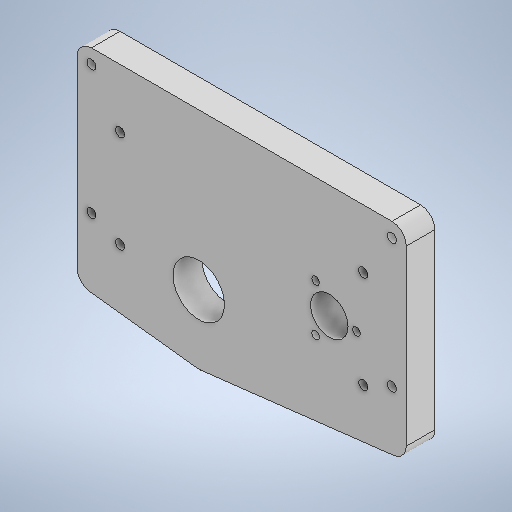
# Autodesk Inventor part: small_plate_motor
Saved by Autodesk Inventor 2025.1 (Build 291241000, 241)
## iProperties
Created: 2024-12-20
Part Number: small_plate_motor
Material: 一般
Document SubType Name: Modeling
Designer: yuki0520
Density: 1 g/cm^3
Appearance: 既定
Author: yuki0520
Autodesk Inventor part; units mm, degrees
ref_plane "YZ Plane" through (0, 0, 0) normal (1, 0, 0) x (0, 1, 0)
ref_plane "XZ Plane" through (0, 0, 0) normal (0, 1, 0) x (-1, 0, 0)
ref_plane "XY Plane" through (0, 0, 0) normal (0, 0, 1) x (1, 0, 0)
sketch "スケッチ1" plane through (0, 0, 0) normal (0, 0, 1) x (1, 0, 0)
  point P0 (0, 0)
sketch "スケッチ2" plane through (0, 0, 0) normal (0, 0, 1) x (1, 0, 0)
  line L0 (72.5, -37.5) -> (-72.5, -37.5)
  line L1 (-72.5, -37.5) -> (-72.5, 37.5)
  line L2 (-72.5, 37.5) -> (72.5, 37.5)
  line L3 (72.5, 37.5) -> (72.5, -37.5)
  line L4 (72.5, -37.5) -> (-72.5, 37.5) construction
  line L5 (-72.5, -37.5) -> (72.5, 37.5) construction
  circle A0 centre (-48, -17) radius 6.05
  circle A1 centre (-48, -17) radius 9
  circle A2 centre (-57, -17) radius 1.6
  circle A3 centre (-48, -26) radius 1.6
  circle A4 centre (-39, -17) radius 1.6
  circle A5 centre (-48, -8) radius 1.6
  line L6 (67.5, 32.5) -> (-67.5, 32.5)
  line L7 (-67.5, 32.5) -> (-67.5, -32.5)
  line L8 (-67.5, -32.5) -> (67.5, -32.5)
  line L9 (67.5, -32.5) -> (67.5, 32.5)
  line L10 (-67.5, 32.5) -> (-67.5, 12.5) construction
  line L11 (-69.1, 32.5) -> (-69.1, 12.5)
  line L12 (-65.9, 12.5) -> (-65.9, 32.5)
  arc A6 (-65.9, 32.5) -> (-69.1, 32.5) centre (-67.5, 32.5) ccw
  arc A7 (-69.1, 12.5) -> (-65.9, 12.5) centre (-67.5, 12.5) ccw
  line L13 (-67.5, 32.5) -> (-47.5, 32.5) construction
  line L14 (-67.5, -32.5) -> (-67.5, -12.5) construction
  line L15 (-65.9, -32.5) -> (-65.9, -12.5)
  line L16 (-69.1, -12.5) -> (-69.1, -32.5)
  arc A8 (-69.1, -32.5) -> (-65.9, -32.5) centre (-67.5, -32.5) ccw
  arc A9 (-65.9, -12.5) -> (-69.1, -12.5) centre (-67.5, -12.5) ccw
  line L17 (-67.5, -32.5) -> (-47.5, -32.5) construction
  line L18 (67.5, 32.5) -> (105, 32.5) construction
  line L19 (-72.5, -17) -> (72.5, -17)
  circle A10 centre (0, -17) radius 9
  circle A11 centre (0, -17) radius 39
  line L20 (-65, 37.5) -> (65, 37.5)
  line L21 (65, 37.5) -> (65, 32.5)
  line L22 (65, 32.5) -> (-65, 32.5)
  line L23 (-65, 32.5) -> (-65, 37.5)
  line L24 (-65, 32.5) -> (0, 0)
  line L25 (0, 0) -> (65, 32.5)
  line L26 (-72.5, 0) -> (72.5, 0)
  line L27 (72.5, 0) -> (72.5, -47.5)
  line L28 (72.5, -47.5) -> (-72.5, -47.5)
  line L29 (-72.5, -47.5) -> (-72.5, 0)
  circle A12 centre (-67.5, 32.5) radius 1.6
  circle A13 centre (-67.5, -12.5) radius 1.6
  line L30 (0, 37.5) -> (0, -47.5)
  line L31 (67.5, 32.5) -> (67.5, 12.5) construction
  line L32 (69.1, 32.5) -> (69.1, 12.5)
  line L33 (65.9, 12.5) -> (65.9, 32.5)
  arc A14 (69.1, 32.5) -> (65.9, 32.5) centre (67.5, 32.5) ccw
  arc A15 (65.9, 12.5) -> (69.1, 12.5) centre (67.5, 12.5) ccw
  line L34 (67.5, -32.5) -> (67.5, -12.5) construction
  line L35 (65.9, -32.5) -> (65.9, -12.5)
  line L36 (69.1, -12.5) -> (69.1, -32.5)
  arc A16 (65.9, -32.5) -> (69.1, -32.5) centre (67.5, -32.5) ccw
  arc A17 (69.1, -12.5) -> (65.9, -12.5) centre (67.5, -12.5) ccw
  circle A18 centre (67.5, 32.5) radius 1.6
  circle A19 centre (67.5, -12.5) radius 1.6
  circle A20 centre (-57.5, -17) radius 1.6
  circle A21 centre (-57.5, 17) radius 1.6
  circle A22 centre (57.5, -17) radius 1.6
  circle A23 centre (57.5, 17) radius 1.6
  circle A24 centre (45.5961, -2) radius 6.55
  circle A25 centre (45.5961, -2) radius 9.5
  circle A26 centre (55.0961, -2) radius 1.35
  circle A27 centre (40.8461, 6.2272) radius 1.35
  circle A28 centre (40.8461, -10.2272) radius 1.35
  circle A29 centre (45.5961, -2) radius 24
  circle A30 centre (0, -17) radius 24
  line L37 (69.5961, -2) -> (21.5961, -2)
  line L38 (0, -41) -> (-72.5, -32.5)
  line L39 (0, -41) -> (72.5, -32.5)
  circle A31 centre (-37.5, -12.5) radius 1.6
  circle A32 centre (-27.5, -17) radius 1.6
  circle A33 centre (-37.5, 32.5) radius 1.6
  circle A34 centre (-27.5, 17) radius 1.6
  line L40 (-42.5, 37.5) -> (-42.5, -47.5)
  circle A35 centre (45.5961, -2) radius 12.2
  point P0 (-67.5, 22.5)
  point P1 (-67.5, -22.5)
  point P2 (-39.1422, -18.5937)
  point P3 (-39.1422, -15.4063)
  point P4 (65, 37.5)
  point P5 (67.5, 22.5)
  point P6 (67.5, -22.5)
  point P7 (-65.9, -12.5)
  point P8 (-69.1, 32.5)
  point P9 (-65, 32.5)
  point P10 (36, -2)
  point P11 (38.741, -15.0124)
  point P12 (33.8387, -0.1107)
  point P13 (63.5912, 34.2414)
  point P14 (65, 36.6)
  point P15 (-65, 36.6)
  point P16 (-63.5912, 34.2414)
  point P17 (-5.5513, -40.3492)
  point P18 (5.5513, -40.3492)
  point P19 (72.5, -32.5)
  point P20 (25.3223, 12.6611)
  point P21 (-25.3223, 12.6611)
  point P22 (-72.5, -32.5)
  point P23 (-42.5, 37.5)
  point P24 (-42.5, -36.0172)
  dimension "d15" = 18
  dimension "d56" = 19
  dimension "d60" = 48
  dimension "d0" = 145
  dimension "d1" = 75
  dimension "d5" = 12.1
  dimension "d16" = 3.2
  dimension "d19" = 360
  dimension "d21" = 5
  dimension "d22" = 20
  dimension "d23" = 90
  dimension "d24" = 3.2
  dimension "d25" = 20
  dimension "d26" = 90
  dimension "d27" = 3.2
  dimension "d36" = 20.5
  dimension "d37" = 18
  dimension "d38" = 78
  dimension "d40" = 48
  dimension "d43" = 130
  dimension "d44" = 65
  dimension "d46" = 47.5
  dimension "d47" = 3.2
  dimension "d48" = 3.2
  dimension "d49" = 10
  dimension "d50" = 10
  dimension "d51" = 17
  dimension "d52" = 17
  dimension "d55" = 13.1
  dimension "d57" = 2.7
  dimension "d58" = 360
  dimension "d59" = 48
  dimension "d62" = 15
  dimension "d65" = 30
  dimension "d70" = 30
  dimension "d71" = 24.4
  constraints: 90 end point, 33 centre point, 18 point on circle, 17 symmetric about line, 13 point on line, 11 parallel, 9 coincident, 9 midpoint, 8 perpendicular, 8 tangent, 7 horizontal, 3 collinear, 2 concentric, 1 horizontal alignment, 45 other
  measures "d0" distance of L1.end L2.end
  measures "d1" distance of L0.end L1.end
  measures "d5" diameter of A0
  measures "d16" diameter of A2
  measures "d21" distance between parallel lines of L2 L6
  measures "d22" distance of L6.end L10.end
  measures "d23" angle of L10 L13
  measures "d24" diameter of A7
  measures "d25" distance of L7.end L14.end
  measures "d26" angle of L17 L14
  measures "d27" diameter of A9
  measures "d36" distance between parallel lines of L0 L19
  measures "d37" diameter of A10
  measures "d38" diameter of A11
  measures "d40" distance of A0.centre A10.centre
  measures "d43" distance of L21.end L22.end
  measures "d44" distance from line of L30.start L23
  measures "d46" distance of L26.end L27.end
  measures "d47" diameter of A20
  measures "d48" diameter of A21
  measures "d49" distance from line of L7 A20.centre
  measures "d50" distance from line of L7 A21.centre
  measures "d51" distance from line of L26 A20.centre
  measures "d52" distance from line of L26 A21.centre
  measures "d55" diameter of A24
  measures "d57" diameter of A26
  measures "d59" diameter of A29
  measures "d62" vertical distance of A11.centre A29.centre
  measures "d65" distance of A13.centre A31.centre
  measures "d70" distance between parallel lines of L1 L40
  measures "d71" diameter of A35
extrude "押し出し1" add sketch "スケッチ2" along normal blind 10 contours L39 A16 L36 L19 L3 | L39 A30 L0 | L0 A30 L8 A11 L39 | A11 L8 A16 L39 | L19 L36 A17 A29 L26 L3 | L39 A16 L8 L9 L19 L36 | A30 L39 L30 L0 | L0 L30 L8 A30 | A11 A29 L19 L35 L8 | L8 A30 L19 A29 A11 | L26 A29 L9 A15 L32 A14 L6 L21 L2 L3 | L19 L9 A19 L36 | L30 L38 A30 L0 | L0 A30 L8 L30 | L8 L30 A10 L19 A30 | L35 L19 L9 L8 | A29 L19 A11 | A11 L19 A22 A29 | A29 L37 L9 L26 | L26 L9 A29 | L19 L35 A29 A19 L9 | A30 L38 L0 | L0 L38 A11 L8 A30 | L8 A30 L19 A10 L30 | A30 A29 L19 | L19 A10 L30 L26 A30 | L38 L40 L8 A11 | L19 A29 L35 | A11 A35 L37 L9 A17 L35 A29 L19 A22 | L19 A29 L37 A35 A11 | L21 L6 L30 L2 | L26 A35 A11 A29 L25 A23 L9 | L9 L37 A35 L26 | A29 A17 L9 L37 | A29 A23 L25 L6 L33 A15 L9 | L8 A11 A4 L19 A32 A30 | A30 L26 A29 | L8 L40 A1 A4 A11 | L35 A19 A29 | A35 L37 A11 A25 | A11 A25 A28 A26 L37 A35 | L30 L6 A33 L40 L2 | L25 A29 A11 L30 L6 | A35 L37 A26 A25 L26 | L26 A25 A27 A11 A35 | A15 L33 A18 L9 | L9 A18 L32 A15 | A30 L26 L30 A10 L19 | L19 A32 A4 A11 A31 L26 A30 | A29 L26 A35 L37 | A30 L25 A11 A29 L26 | L26 L25 A30 | A11 L19 A4 | A4 A1 A11 | A25 A11 | A11 A25 L37 A24 A26 A28 | A35 L26 A11 L37 | L30 A11 L24 L40 L6 A33 | L25 A29 | A25 A26 L37 A24 L26 | L26 A24 A25 A27 | A35 L26 A29 A11 | A11 L26 A35 | A30 L24 L26 | L26 A11 L24 A30 | L30 A30 L25 | L24 A30 L30 | A30 L30 A11 L25 | L40 A0 L19 A4 A1 | A4 L19 A1 | L19 A11 A4 | L19 A4 A1 | A1 A4 A11 | A11 L37 A25 | A11 L26 A25 L37 | L30 A30 L24 A11 | A29 A11 L25 | L26 L40 L24 A11 | A11 A31 A4 A1 L40 L26 | L40 L19 A0 | L19 A0 L40 A1 A4 | A25 L26 A24 L37 | L19 L40 A0 picked at (-42.3988, -18.41) picked at (-42.3988, -15.59)
fillet "フィレット1" radius 5 5 edges at (72.5, 37.5, 5) (72.5, -32.5, 5) (0, -41, 5) (-42.5, 37.5, 5) (-42.5, -36.0172, 5)
equation "\"d25\" = d22"
equation "\"d27\" = d24"
equation "\"d40\" = d39"
equation "\"d44\" = 0.5 * d43"
equation "\"d39\" = 48"
